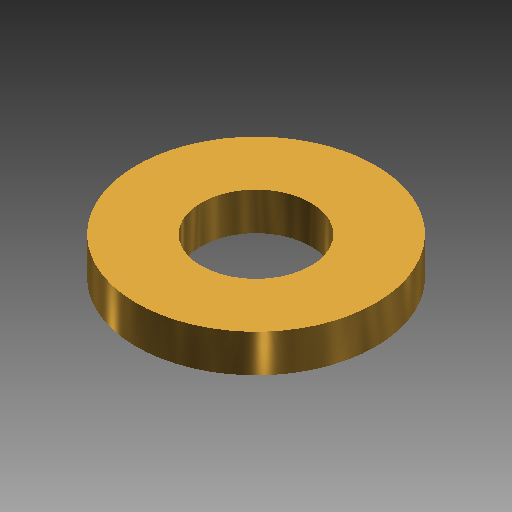
# Autodesk Inventor part: 312-04
Saved by Autodesk Inventor 2019 (Build 230136000, 136)
## iProperties
Company: Autodesk Inc.
Created: 2007-10-25
Part Number: 312-04
Document SubType Name: Modeling
Designer: Autodesk Inc.
Density: 7.85 g/cm^3
Mass: 5.27713 g
Surface Area: 7.0923 cm^2
Volume: 0.672246 cm^3
Material: Steel
Description: SHIM 8.7 MM X 3 MM
Appearance: Brass - Satin
Component Category: Fasteners
Author: Inventor
Autodesk Inventor part; units mm, degrees
ref_plane "YZ Plane" through (0, 0, 0) normal (1, 0, 0) x (0, 1, 0)
ref_plane "XZ Plane" through (0, 0, 0) normal (0, 1, 0) x (-1, 0, 0)
ref_plane "XY Plane" through (0, 0, 0) normal (0, 0, 1) x (1, 0, 0)
sketch "Sketch1" plane through (0, 0, 0) normal (0, 0, 1) x (1, 0, 0)
  line L0 (0, -2.1) -> (0, 2.1) projected
  line L1 (-1.9, 0) -> (11.4, 0) projected
  line L2 (4.35, 1.5) -> (4.35, -1.5)
  line L3 (4.35, -1.5) -> (9.5, -1.5)
  line L4 (9.5, -1.5) -> (9.5, 1.5)
  line L5 (9.5, 1.5) -> (4.35, 1.5)
  point P0 (0, 0)
  point P1 (9.5, 0)
  dimension "d0" = 8.7
  dimension "d1" = 19
  dimension "d2" = 3
  constraints: 8 end point, 2 parallel, 2 perpendicular, 1 midpoint, 1 point on line
  measures "d0" diameter of L2 L0
  measures "d1" diameter of L4 L0
  measures "d2" distance between parallel lines of L3 L5
revolve "Revolution1" add sketch "Sketch1" angle 360 about axis through (0, -10, 0) along (0, 1, 0)
body "Solid1"
